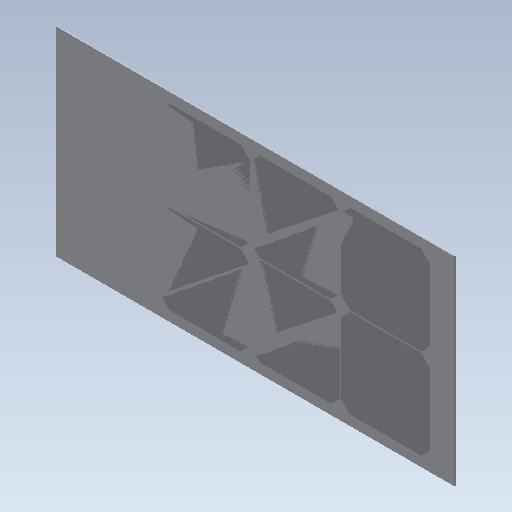
# Autodesk Inventor part: solar1
Saved by Autodesk Inventor 2020 (Build 240168000, 168)
## iProperties
Created: 2016-11-10
Part Number: solar1
Material: Aluminum 6061-AHC
Document SubType Name: Modeling
Designer: jous
Density: 2.71 g/cm^3
Appearance: Aluminum - Dark
Mass: 816.658 g
Surface Area: 3173.37 cm^2
Volume: 301.35 cm^3
Author: jous
Autodesk Inventor part; units mm, degrees
ref_plane "YZ Plane" through (0, 0, 0) normal (1, 0, 0) x (0, 1, 0)
ref_plane "XZ Plane" through (0, 0, 0) normal (0, 1, 0) x (-1, 0, 0)
ref_plane "XY Plane" through (0, 0, 0) normal (0, 0, 1) x (1, 0, 0)
sketch "Sketch1" plane through (0, 0, 0) normal (0, 0, 1) x (1, 0, 0)
  line L0 (-400, -140) -> (160, -140)
  line L1 (160, -140) -> (160, 140)
  line L2 (160, 140) -> (-400, 140)
  line L3 (-400, 140) -> (-400, -140)
  point P0 (0, 0)
  dimension "d0" = 560
  dimension "d1" = 280
  dimension "d36" = 400
  constraints: 8 end point, 2 parallel, 1 horizontal, 1 perpendicular
  measures "d0" distance of L2.end L1.end
  measures "d1" distance of L1.end L0.end
  measures "d36" distance from line of L3 point (0, 0)
sketch "Sketch4" plane through (0, 0, 0) normal (0, 0, 1) x (1, 0, 0)
  line L0 (-380, -1) -> (-367.5, -1)
  line L1 (-255, -1) -> (-255, -13.5)
  line L2 (-255, -126) -> (-267.5, -126)
  line L3 (-380, -126) -> (-380, -113.5)
  line L4 (-380, -13.5) -> (-367.5, -1)
  line L5 (-267.5, -1) -> (-255, -13.5)
  line L6 (-255, -113.5) -> (-267.5, -126)
  line L7 (-367.5, -126) -> (-380, -113.5)
  line L8 (-367.5, -1) -> (-267.5, -1)
  line L9 (-380, -13.5) -> (-380, -1)
  line L10 (-267.5, -1) -> (-255, -1)
  line L11 (-255, -13.5) -> (-255, -113.5)
  line L12 (-267.5, -126) -> (-367.5, -126)
  line L13 (-255, -113.5) -> (-255, -126)
  line L14 (-367.5, -126) -> (-380, -126)
  line L15 (-380, -113.5) -> (-380, -13.5)
  line L16 (-400, -140) -> (160, -140) projected
  line L17 (-400, 140) -> (-400, -140) projected
  point P0 (0, 0)
  dimension "d6" = 125
  dimension "d7" = 125
  dimension "d8" = 12.5
  dimension "d9" = 12.5
  dimension "d10" = 12.5
  dimension "d11" = 12.5
  dimension "d12" = 12.5
  dimension "d13" = 12.5
  dimension "d14" = 12.5
  dimension "d15" = 12.5
  dimension "d22" = 14
  dimension "d23" = 20
  constraints: 32 end point, 18 parallel, 9 perpendicular, 3 horizontal, 3 point on line
  measures "d6" distance of L2.start L3.start
  measures "d7" distance of L1.start L2.start
  measures "d8" distance of L0.end L0.start
  measures "d9" distance of L1.start L5.start
  measures "d10" distance of L1.end L1.start
  measures "d11" distance of L2.start L6.start
  measures "d12" distance of L2.end L2.start
  measures "d13" distance of L3.start L7.start
  measures "d14" distance of L3.end L3.start
  measures "d15" distance of L4.start L0.start
  measures "d22" distance between parallel lines of L12 L16
  measures "d23" distance between parallel lines of L15 L17
sketch "Sketch5" plane through (0, 0, 0) normal (0, 0, 1) x (1, 0, 0)
  line L0 (-380, -13.5) -> (-367.5, -1) projected
  line L1 (-367.5, -1) -> (-267.5, -1) projected
  line L2 (-267.5, -1) -> (-255, -13.5) projected
  line L3 (-255, -13.5) -> (-255, -113.5) projected
  line L4 (-267.5, -126) -> (-367.5, -126) projected
  line L5 (-255, -113.5) -> (-267.5, -126) projected
  line L6 (-367.5, -126) -> (-380, -113.5) projected
  line L7 (-380, -113.5) -> (-380, -13.5) projected
  point P0 (0, 0)
boundary_patch "Boundary Patch3"
pattern_linear "Rectangular Pattern1" count 4 spacing 127 along (1, 0, 0) count 2 spacing 127 along (0, 1, 0) of "Boundary Patch3"
sketch "Sketch6" plane through (0, 0, 0) normal (0, 0, 1) x (1, 0, 0)
  line L0 (160, 140) -> (-400, 140) projected
  line L1 (-400, 140) -> (-400, -140) projected
  line L2 (-400, -140) -> (160, -140) projected
  line L3 (160, -140) -> (160, 140) projected
  line L4 (-367.5, 126) -> (-267.5, 126) projected
  line L5 (-240.5, 126) -> (-140.5, 126) projected
  line L6 (-253, 113.5) -> (-240.5, 126) projected
  line L7 (-267.5, 126) -> (-255, 113.5) projected
  line L8 (-380, 13.5) -> (-380, 113.5) projected
  line L9 (-380, 113.5) -> (-367.5, 126) projected
  line L10 (-367.5, 1) -> (-380, 13.5) projected
  line L11 (-267.5, 1) -> (-367.5, 1) projected
  line L12 (-255, 113.5) -> (-255, 13.5) projected
  line L13 (-255, 13.5) -> (-267.5, 1) projected
  line L14 (-240.5, 1) -> (-253, 13.5) projected
  line L15 (-253, 13.5) -> (-253, 113.5) projected
  line L16 (-128, 113.5) -> (-128, 13.5) projected
  line L17 (-126, 13.5) -> (-126, 113.5) projected
  line L18 (-140.5, 126) -> (-128, 113.5) projected
  line L19 (-126, 113.5) -> (-113.5, 126) projected
  line L20 (-113.5, 126) -> (-13.5, 126) projected
  line L21 (-13.5, 126) -> (-1, 113.5) projected
  line L22 (1, 113.5) -> (13.5, 126) projected
  line L23 (13.5, 126) -> (113.5, 126) projected
  line L24 (113.5, 126) -> (126, 113.5) projected
  line L25 (126, 113.5) -> (126, 13.5) projected
  line L26 (1, 13.5) -> (1, 113.5) projected
  line L27 (-1, 113.5) -> (-1, 13.5) projected
  line L28 (-380, -113.5) -> (-380, -13.5) projected
  line L29 (-380, -13.5) -> (-367.5, -1) projected
  line L30 (-267.5, -1) -> (-255, -13.5) projected
  line L31 (-367.5, -1) -> (-267.5, -1) projected
  line L32 (-253, -13.5) -> (-240.5, -1) projected
  line L33 (-140.5, -1) -> (-128, -13.5) projected
  line L34 (-240.5, -1) -> (-140.5, -1) projected
  line L35 (-140.5, 1) -> (-240.5, 1) projected
  line L36 (-128, 13.5) -> (-140.5, 1) projected
  line L37 (13.5, 1) -> (1, 13.5) projected
  line L38 (-1, 13.5) -> (-13.5, 1) projected
  line L39 (-113.5, 1) -> (-126, 13.5) projected
  line L40 (126, 13.5) -> (113.5, 1) projected
  line L41 (113.5, 1) -> (13.5, 1) projected
  line L42 (13.5, -1) -> (113.5, -1) projected
  line L43 (-13.5, 1) -> (-113.5, 1) projected
  line L44 (-113.5, -1) -> (-13.5, -1) projected
  line L45 (-126, -13.5) -> (-113.5, -1) projected
  line L46 (-13.5, -1) -> (-1, -13.5) projected
  line L47 (1, -13.5) -> (13.5, -1) projected
  line L48 (113.5, -1) -> (126, -13.5) projected
  line L49 (-267.5, -126) -> (-367.5, -126) projected
  line L50 (-255, -13.5) -> (-255, -113.5) projected
  line L51 (-253, -113.5) -> (-253, -13.5) projected
  line L52 (-128, -13.5) -> (-128, -113.5) projected
  line L53 (-126, -113.5) -> (-126, -13.5) projected
  line L54 (-1, -13.5) -> (-1, -113.5) projected
  line L55 (1, -113.5) -> (1, -13.5) projected
  line L56 (126, -13.5) -> (126, -113.5) projected
  line L57 (126, -113.5) -> (113.5, -126) projected
  line L58 (113.5, -126) -> (13.5, -126) projected
  line L59 (13.5, -126) -> (1, -113.5) projected
  line L60 (-1, -113.5) -> (-13.5, -126) projected
  line L61 (-13.5, -126) -> (-113.5, -126) projected
  line L62 (-113.5, -126) -> (-126, -113.5) projected
  line L63 (-128, -113.5) -> (-140.5, -126) projected
  line L64 (-140.5, -126) -> (-240.5, -126) projected
  line L65 (-240.5, -126) -> (-253, -113.5) projected
  line L66 (-255, -113.5) -> (-267.5, -126) projected
  line L67 (-367.5, -126) -> (-380, -113.5) projected
  point P0 (0, 0)
sketch "Sketch9" plane through (0, 0, 0) normal (0, 0, 1) x (1, 0, 0)
  line L0 (-367.5, 126) -> (-267.5, 126)
  line L1 (-240.5, 126) -> (-140.5, 126)
  line L2 (-253, 113.5) -> (-240.5, 126)
  line L3 (-267.5, 126) -> (-255, 113.5)
  line L4 (-380, 13.5) -> (-380, 113.5)
  line L5 (-380, 113.5) -> (-367.5, 126)
  line L6 (-367.5, 1) -> (-380, 13.5)
  line L7 (-267.5, 1) -> (-367.5, 1)
  line L8 (-255, 113.5) -> (-255, 13.5)
  line L9 (-255, 13.5) -> (-267.5, 1)
  line L10 (-240.5, 1) -> (-253, 13.5)
  line L11 (-253, 13.5) -> (-253, 113.5)
  line L12 (-128, 113.5) -> (-128, 13.5)
  line L13 (-126, 13.5) -> (-126, 113.5)
  line L14 (-140.5, 126) -> (-128, 113.5)
  line L15 (-126, 113.5) -> (-113.5, 126)
  line L16 (-113.5, 126) -> (-13.5, 126)
  line L17 (-13.5, 126) -> (-1, 113.5)
  line L18 (1, 113.5) -> (13.5, 126)
  line L19 (13.5, 126) -> (113.5, 126)
  line L20 (113.5, 126) -> (126, 113.5)
  line L21 (126, 113.5) -> (126, 13.5)
  line L22 (1, 13.5) -> (1, 113.5)
  line L23 (-1, 113.5) -> (-1, 13.5)
  line L24 (-380, -113.5) -> (-380, -13.5)
  line L25 (-380, -13.5) -> (-367.5, -1)
  line L26 (-267.5, -1) -> (-255, -13.5)
  line L27 (-367.5, -1) -> (-267.5, -1)
  line L28 (-253, -13.5) -> (-240.5, -1)
  line L29 (-140.5, -1) -> (-128, -13.5)
  line L30 (-240.5, -1) -> (-140.5, -1)
  line L31 (-140.5, 1) -> (-240.5, 1)
  line L32 (-128, 13.5) -> (-140.5, 1)
  line L33 (13.5, 1) -> (1, 13.5)
  line L34 (-1, 13.5) -> (-13.5, 1)
  line L35 (-113.5, 1) -> (-126, 13.5)
  line L36 (126, 13.5) -> (113.5, 1)
  line L37 (113.5, 1) -> (13.5, 1)
  line L38 (13.5, -1) -> (113.5, -1)
  line L39 (-13.5, 1) -> (-113.5, 1)
  line L40 (-113.5, -1) -> (-13.5, -1)
  line L41 (-126, -13.5) -> (-113.5, -1)
  line L42 (-13.5, -1) -> (-1, -13.5)
  line L43 (1, -13.5) -> (13.5, -1)
  line L44 (113.5, -1) -> (126, -13.5)
  line L45 (-267.5, -126) -> (-367.5, -126)
  line L46 (-255, -13.5) -> (-255, -113.5)
  line L47 (-253, -113.5) -> (-253, -13.5)
  line L48 (-128, -13.5) -> (-128, -113.5)
  line L49 (-126, -113.5) -> (-126, -13.5)
  line L50 (-1, -13.5) -> (-1, -113.5)
  line L51 (1, -113.5) -> (1, -13.5)
  line L52 (126, -13.5) -> (126, -113.5)
  line L53 (126, -113.5) -> (113.5, -126)
  line L54 (113.5, -126) -> (13.5, -126)
  line L55 (13.5, -126) -> (1, -113.5)
  line L56 (-1, -113.5) -> (-13.5, -126)
  line L57 (-13.5, -126) -> (-113.5, -126)
  line L58 (-113.5, -126) -> (-126, -113.5)
  line L59 (-128, -113.5) -> (-140.5, -126)
  line L60 (-140.5, -126) -> (-240.5, -126)
  line L61 (-240.5, -126) -> (-253, -113.5)
  line L62 (-255, -113.5) -> (-267.5, -126)
  line L63 (-367.5, -126) -> (-380, -113.5)
  point P0 (0, 0)
  point P1 (0, 0)
  constraints: 128 end point
extrude "Extrusion4" add sketch "Sketch6" against normal blind 2
extrude "Extrusion6" add sketch "Sketch9" against normal blind 1.9
equation "\"d9\" = d8"
equation "\"d10\" = d9"
equation "\"d11\" = d10"
equation "\"d12\" = d11"
equation "\"d13\" = d12"
equation "\"d14\" = d13"
equation "\"d15\" = d8"
body "Solid4"
body "Srf3"
body "Srf4"
body "Srf5"
body "Srf6"
body "Srf8"
body "Srf9"
body "Srf10"
body "Srf11"
